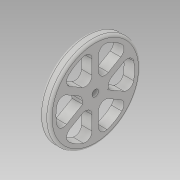
# Autodesk Inventor part: Wheel
Saved by Autodesk Inventor 2019 (Build 230136000, 136)
## iProperties
Created: 2020-03-03
Part Number: Wheel
Material: Genérico
Document SubType Name: Modeling
Designer: daniel.regner
Density: 1 g/cm^3
Appearance: Padrão
Author: daniel.regner
Autodesk Inventor part; units mm, degrees
ref_plane "YZ Plane" through (0, 0, 0) normal (1, 0, 0) x (0, 1, 0)
ref_plane "XZ Plane" through (0, 0, 0) normal (0, 1, 0) x (-1, 0, 0)
ref_plane "XY Plane" through (0, 0, 0) normal (0, 0, 1) x (1, 0, 0)
sketch "Esboço1" plane through (0, 0, 0) normal (1, 0, 0) x (0, 1, 0)
  circle A0 centre (0, 0) radius 35
  circle A1 centre (0, 0) radius 2.5
  line L0 (9.6825, 2.5) -> (29.8957, 2.5)
  line L1 (29.8957, -2.5) -> (9.6825, -2.5)
  line L2 (17.1129, 24.6404) -> (7.0063, 7.1353)
  line L3 (2.6762, 9.6353) -> (12.7828, 27.1404)
  line L4 (-12.7828, 27.1404) -> (-2.6762, 9.6353)
  line L5 (-7.0063, 7.1353) -> (-17.1129, 24.6404)
  line L6 (-29.8957, 2.5) -> (-9.6825, 2.5)
  line L7 (-9.6825, -2.5) -> (-29.8957, -2.5)
  line L8 (-17.1129, -24.6404) -> (-7.0063, -7.1353)
  line L9 (-2.6762, -9.6353) -> (-12.7828, -27.1404)
  line L10 (12.7828, -27.1404) -> (2.6762, -9.6353)
  line L11 (7.0063, -7.1353) -> (17.1129, -24.6404)
  arc A2 (29.8957, 2.5) -> (17.1129, 24.6404) centre (0, 0) ccw
  arc A3 (12.7828, 27.1404) -> (-12.7828, 27.1404) centre (0, 0) ccw
  arc A4 (-17.1129, 24.6404) -> (-29.8957, 2.5) centre (0, 0) ccw
  arc A5 (-29.8957, -2.5) -> (-17.1129, -24.6404) centre (0, 0) ccw
  arc A6 (-12.7828, -27.1404) -> (12.7828, -27.1404) centre (0, 0) ccw
  arc A7 (17.1129, -24.6404) -> (29.8957, -2.5) centre (0, 0) ccw
  arc A8 (-2.6762, -9.6353) -> (2.6762, -9.6353) centre (0, 0) ccw
  arc A9 (2.6762, 9.6353) -> (-2.6762, 9.6353) centre (0, 0) ccw
  arc A10 (7.0063, -7.1353) -> (9.6825, -2.5) centre (0, 0) ccw
  arc A11 (9.6825, 2.5) -> (7.0063, 7.1353) centre (0, 0) ccw
  arc A12 (-7.0063, 7.1353) -> (-9.6825, 2.5) centre (0, 0) ccw
  arc A13 (-9.6825, -2.5) -> (-7.0063, -7.1353) centre (0, 0) ccw
  dimension "d0" = 70
  dimension "d3" = 5
  dimension "d4" = 5
  dimension "d5" = 2.5
  dimension "d8" = 360
  dimension "d10" = 30
  dimension "d11" = 10
  constraints: 24 end point, 24 point on circle, 14 centre point, 3 coincident, 1 horizontal, 1 parallel, 37 other
  measures "d0" diameter of A0
  measures "d3" diameter of A1
  measures "d4" distance between parallel lines of L1 L0
  measures "d5" distance from line of point (0, 0) L0
  measures "d10" radius of A7
  measures "d11" radius of A11
extrude "Extrusão1" add sketch "Esboço1" along normal mid plane 8
fillet "Arredondamento1" radius 2 2 edges at (-4, -35, 0) (4, -35, 0)
fillet "Arredondamento2" radius 5 44 edges at (2, 12.7828, -27.1404) (-2, 12.7828, -27.1404) (2, 17.1129, -24.6404) (-2, 17.1129, -24.6404) (2, 29.8957, 2.5) (-2, 29.8957, 2.5) (2, 29.8957, -2.5) (-2, 29.8957, -2.5) (2, 2.6762, -9.6353) (-2, 2.6762, -9.6353) (2, 7.0063, -7.1353) (-2, 7.0063, -7.1353) (2, 9.6825, -2.5) (-2, 9.6825, -2.5) (2, 9.6825, 2.5) (-2, 9.6825, 2.5) (2, 7.0063, 7.1353) (-2, 7.0063, 7.1353) (2, 17.1129, 24.6404) (-2, 17.1129, 24.6404) (2, 12.7828, 27.1404) (-2, 12.7828, 27.1404) (2, -7.0063, 7.1353) (-2, -7.0063, 7.1353) (2, -9.6825, 2.5) (-2, -9.6825, 2.5) (2, 2.6762, 9.6353) (-2, 2.6762, 9.6353) (2, -7.0063, -7.1353) (-2, -7.0063, -7.1353) (2, -9.6825, -2.5) (-2, -9.6825, -2.5) (2, -12.7828, 27.1404) (-2, -12.7828, 27.1404) (2, -17.1129, 24.6404) (-2, -17.1129, 24.6404) (2, -29.8957, -2.5) (-2, -29.8957, -2.5) (2, -29.8957, 2.5) (-2, -29.8957, 2.5) (2, -12.7828, -27.1404) (-2, -12.7828, -27.1404) (2, -17.1129, -24.6404) (-2, -17.1129, -24.6404)
equation "\"d5\" = 0.5 * d4"
